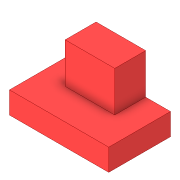
# Autodesk Inventor part: BOB-10031 USB Micro B Breakout
Saved by Autodesk Inventor 2018.3 (Build 223284000, 284)
## iProperties
Created: 2018-12-11
Part Number: BOB-10031 USB Micro B Breakout
Material: Generic
Document SubType Name: Modeling
Designer: tei06398
Mass: 2.61081 g
Surface Area: 14.5067 cm^2
Volume: 2.61081 cm^3
Density: 1 g/cm^3
Appearance: Default
Author: tei06398
Autodesk Inventor part; units mm, degrees
ref_plane "YZ Plane" through (0, 0, 0) normal (1, 0, 0) x (0, 1, 0)
ref_plane "XZ Plane" through (0, 0, 0) normal (0, 1, 0) x (-1, 0, 0)
ref_plane "XY Plane" through (0, 0, 0) normal (0, 0, 1) x (1, 0, 0)
sketch "Sketch1" plane through (0, 0, 0) normal (0, 0, 1) x (1, 0, 0)
  line L0 (0, 0) -> (23.54, 0)
  line L1 (23.54, 0) -> (23.54, 14.75)
  line L2 (23.54, 14.75) -> (0, 14.75)
  line L3 (0, 14.75) -> (0, 0)
  dimension "d0" = 23.54
  dimension "d1" = 14.75
  constraints: 8 end point, 2 parallel, 1 horizontal, 1 perpendicular
  measures "d0" distance of L2.end L1.end
  measures "d1" distance of L1.end L0.end
extrude "Extrusion1" add sketch "Sketch1" against normal blind 14.65
sketch "Sketch2" plane through (0, 14.75, 0) normal (0, 1, 0) x (1, 0, 0)
  line L0 (23.54, 0) -> (0, 0) projected
  line L1 (0, 0) -> (0, 14.65) projected
  line L2 (23.54, 14.65) -> (0, 14.65) projected
  line L3 (0, 0) -> (5.8865, 0)
  line L4 (5.8865, 0) -> (5.8865, 14.65)
  line L5 (5.8865, 14.65) -> (0, 14.65)
  line L6 (0, 14.65) -> (0, 0)
  line L7 (23.54, 14.65) -> (17.6472, 14.65)
  line L8 (17.6472, 14.65) -> (17.6472, 0)
  line L9 (17.6472, 0) -> (23.54, 0)
  line L10 (23.54, 0) -> (23.54, 14.65)
  line L11 (5.8865, 0) -> (17.6472, 0)
  line L12 (17.6472, 0) -> (17.6472, 7.325)
  line L13 (17.6472, 7.325) -> (5.8865, 7.325)
  line L14 (5.8865, 7.325) -> (5.8865, 0)
  dimension "d4" = 5.8864
  dimension "d5" = 5.8928
  constraints: 24 end point, 6 parallel, 3 horizontal, 3 perpendicular, 2 point on line, 1 midpoint
  measures "d4" distance of L5.end L4.end
  measures "d5" distance of L9.end L8.end
extrude "Extrusion2" cut sketch "Sketch2" against normal blind 9.57 contours L0 L8 L2 L10 | L0 L4 L13 L8 | L0 L1 L2 L4
body "Solid1"
